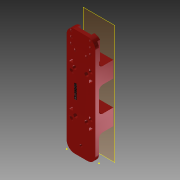
# Autodesk Inventor part: 150mm Link_V2 PART A
Saved by Autodesk Inventor 2015 (Build 190159000, 159)
## iProperties
Created: 2016-11-30
Part Number: 150mm Link_V2 PART A
Material: Generic
Document SubType Name: Modeling
Designer: Rudge-Top
Density: 1 g/cm^3
Appearance: Orange-Red
Author: Rudge-Top
Autodesk Inventor part; units mm, degrees
ref_plane "YZ Plane" through (0, 0, 0) normal (1, 0, 0) x (0, 1, 0)
ref_plane "XZ Plane" through (0, 0, 0) normal (0, 1, 0) x (-1, 0, 0)
ref_plane "XY Plane" through (0, 0, 0) normal (0, 0, 1) x (1, 0, 0)
sketch "Sketch1" plane through (0, 0, 0) normal (1, 0, 0) x (0, 1, 0)
  line L0 (120, 0) -> (150, 0)
  line L1 (150, 0) -> (150, -40)
  line L2 (150, -40) -> (120, -40)
  line L3 (150, 5) -> (0, 5)
  line L4 (0, -45) -> (150, -45)
  line L5 (150, 0) -> (150, 5)
  line L6 (150, -40) -> (150, -45)
  line L7 (0, -40) -> (0, -45)
  line L8 (0, 0) -> (0, 5)
  line L9 (115, -5) -> (115, -35)
  arc A0 (120, 0) -> (115, -5) centre (120, -5) ccw
  arc A1 (115, -35) -> (120, -40) centre (120, -35) ccw
  line L10 (87.5, 0) -> (62.5, 0)
  line L11 (57.5, -5) -> (57.5, -35)
  line L12 (62.5, -40) -> (87.5, -40)
  line L13 (92.5, -35) -> (92.5, -5)
  arc A2 (87.5, -40) -> (92.5, -35) centre (87.5, -35) ccw
  arc A3 (57.5, -35) -> (62.5, -40) centre (62.5, -35) ccw
  arc A4 (62.5, 0) -> (57.5, -5) centre (62.5, -5) ccw
  arc A5 (92.5, -5) -> (87.5, 0) centre (87.5, -5) ccw
  line L14 (0, 0) -> (30, 0)
  line L15 (35, -5) -> (35, -35)
  line L16 (30, -40) -> (0, -40)
  arc A6 (35, -5) -> (30, 0) centre (30, -5) ccw
  arc A7 (30, -40) -> (35, -35) centre (30, -35) ccw
  point P0 (57.5, -40)
  point P1 (92.5, -40)
  point P2 (35, 0)
  dimension "d1" = 150
  dimension "d2" = 40
  dimension "d3" = 90
  dimension "d4" = 5
  dimension "d5" = 35
  dimension "d6" = 5
  dimension "d7" = 35
  dimension "d8" = 5
  dimension "d9" = 22.5
  dimension "d10" = 5
  dimension "d11" = 35
  dimension "d12" = 5
  constraints: 34 end point, 16 point on circle, 16 tangent, 9 point on line, 8 centre point, 8 perpendicular, 5 equal radius, 3 horizontal, 2 parallel
  measures "d1" distance of L8.start L0.end
  measures "d2" distance of L0.end L1.end
  measures "d3" angle of L0 L1
  measures "d4" distance between parallel lines of L0 L3
  measures "d5" distance between parallel lines of L1 L9
  measures "d6" radius of A0
  measures "d7" distance of point (92.5, -40) point (57.5, -40)
  measures "d8" distance between parallel lines of L3 L10
  measures "d9" distance between parallel lines of L13 L9
  measures "d10" radius of A2
  measures "d11" distance of L8.start point (35, 0)
  measures "d12" radius of A6
extrude "Extrusion1" add sketch "Sketch1" along normal blind 40 contours A0 L9 A1 L2 L6 L4 L7 L16 A7 L15 A6 L14 L8 L3 L5 L0
sketch "Sketch2" plane through (40, 0, 0) normal (1, 0, 0) x (0, 0, -1)
  arc A0 (35, 57.5) -> (40, 62.5) centre (35, 62.5) ccw projected
  line L0 (35, 57.5) -> (5, 57.5) projected
  arc A1 (0, 62.5) -> (5, 57.5) centre (5, 62.5) ccw projected
  line L1 (0, 62.5) -> (0, 87.5) projected
  arc A2 (5, 92.5) -> (0, 87.5) centre (5, 87.5) ccw projected
  line L2 (5, 92.5) -> (35, 92.5) projected
  arc A3 (40, 87.5) -> (35, 92.5) centre (35, 87.5) ccw projected
  line L3 (40, 87.5) -> (40, 62.5) projected
  line L4 (0, 0) -> (0, 30) projected
  arc A4 (5, 35) -> (0, 30) centre (5, 30) ccw projected
  line L5 (5, 35) -> (35, 35) projected
  arc A5 (40, 30) -> (35, 35) centre (35, 30) ccw projected
  line L6 (40, 30) -> (40, 0) projected
  line L7 (40, 0) -> (45, 0) projected
  line L8 (45, 0) -> (45, 150) projected
  line L9 (45, 150) -> (40, 150) projected
  line L10 (40, 150) -> (40, 120) projected
  arc A6 (35, 115) -> (40, 120) centre (35, 120) ccw projected
  line L11 (35, 115) -> (5, 115) projected
  arc A7 (0, 120) -> (5, 115) centre (5, 120) ccw projected
  line L12 (0, 120) -> (0, 150) projected
  line L13 (0, 150) -> (-5, 150) projected
  line L14 (-5, 150) -> (-5, 0) projected
  line L15 (-5, 0) -> (0, 0) projected
  circle A8 centre (35, 45.25) radius 2.5
  circle A9 centre (25, 45.25) radius 2.5
  circle A10 centre (15, 45.25) radius 2.5
  circle A11 centre (5, 45.25) radius 2.5
  circle A12 centre (35, 104.75) radius 2.5
  circle A13 centre (25, 104.75) radius 2.5
  circle A14 centre (15, 104.75) radius 2.5
  circle A15 centre (5, 104.75) radius 2.5
  dimension "d15" = 5
  dimension "d16" = 5
  dimension "d17" = 5
  dimension "d18" = 5
  dimension "d19" = 10
  dimension "d20" = 20
  dimension "d21" = 30
  dimension "d22" = 40
  dimension "d23" = 5
  dimension "d24" = 5
  dimension "d25" = 5
  dimension "d26" = 5
  dimension "d27" = 12.25
  dimension "d28" = 12.25
  dimension "d29" = 12.25
  dimension "d30" = 12.25
  dimension "d31" = 12.25
  dimension "d32" = 12.25
  dimension "d33" = 12.25
  dimension "d34" = 12.25
  constraints: 8 centre point
  measures "d15" diameter of A8
  measures "d16" diameter of A9
  measures "d17" diameter of A10
  measures "d18" diameter of A11
  measures "d19" distance from line of L14 A11.centre
  measures "d20" distance from line of A10.centre L14
  measures "d21" distance from line of A9.centre L14
  measures "d22" distance from line of A8.centre L14
  measures "d23" diameter of A12
  measures "d24" diameter of A13
  measures "d25" diameter of A14
  measures "d26" diameter of A15
  measures "d27" distance from line of A12.centre L2
  measures "d28" distance from line of L2 A13.centre
  measures "d29" distance from line of L2 A14.centre
  measures "d30" distance from line of L2 A15.centre
  measures "d31" distance from line of A8.centre L0
  measures "d32" distance from line of A9.centre L0
  measures "d33" distance from line of A10.centre L0
  measures "d34" distance from line of A11.centre L0
fillet "Fillet1" radius 11 8 edges at (40, 0, 2.5) (0, 0, 2.5) (40, 0, -42.5) (0, 0, -42.5) (40, 150, 2.5) (40, 150, -42.5) (0, 150, -42.5) (0, 150, 2.5)
sketch "Sketch3" plane through (0, 11, -45) normal (0, 0, -1) x (-1, 0, 0)
  line L0 (0, 51.5) -> (-40, 51.5) projected
  arc A0 (0, 128) -> (-11, 139) centre (-11, 128) ccw projected
  line L1 (-11, 139) -> (-29, 139) projected
  arc A1 (-29, 139) -> (-40, 128) centre (-29, 128) ccw projected
  line L2 (-40, 0) -> (-40, 128) projected
  arc A2 (-40, 0) -> (-29, -11) centre (-29, 0) ccw projected
  line L3 (-11, -11) -> (-29, -11) projected
  arc A3 (-11, -11) -> (0, 0) centre (-11, 0) ccw projected
  line L4 (0, 0) -> (0, 128) projected
  line L5 (-40, 51.5) -> (-40, 46.5) projected
  line L6 (-40, 46.5) -> (-40, 51.5) projected
  line L7 (-40, 51.5) -> (-40, 76.5) projected
  line L8 (-40, 76.5) -> (-40, 81.5) projected
  line L9 (-40, 81.5) -> (-40, 76.5) projected
  line L10 (-40, 76.5) -> (-40, 51.5) projected
  line L11 (-40, 128) -> (-40, 109) projected
  line L12 (-40, 109) -> (-40, 104) projected
  line L13 (-40, 104) -> (-40, 109) projected
  line L14 (-40, 109) -> (-40, 128) projected
  line L15 (-40, 128) -> (-40, 0) projected
  line L16 (-40, 0) -> (-40, 19) projected
  line L17 (-40, 19) -> (-40, 24) projected
  line L18 (-40, 24) -> (-40, 19) projected
  line L19 (-40, 19) -> (-40, 0) projected
  line L20 (-40, 0) -> (-40, 128) projected
  line L21 (-9, 26.5) -> (-31, 26.5)
  line L22 (-36, 31.5) -> (-36, 39)
  line L23 (-31, 44) -> (-9, 44)
  line L24 (-4, 39) -> (-4, 31.5)
  arc A4 (-36, 31.5) -> (-31, 26.5) centre (-31, 31.5) ccw
  arc A5 (-31, 44) -> (-36, 39) centre (-31, 39) ccw
  arc A6 (-4, 39) -> (-9, 44) centre (-9, 39) ccw
  arc A7 (-9, 26.5) -> (-4, 31.5) centre (-9, 31.5) ccw
  line L25 (-9, 84) -> (-31, 84)
  line L26 (-36, 89) -> (-36, 96.5)
  line L27 (-31, 101.5) -> (-9, 101.5)
  line L28 (-4, 96.5) -> (-4, 89)
  arc A8 (-36, 89) -> (-31, 84) centre (-31, 89) ccw
  arc A9 (-31, 101.5) -> (-36, 96.5) centre (-31, 96.5) ccw
  arc A10 (-4, 96.5) -> (-9, 101.5) centre (-9, 96.5) ccw
  arc A11 (-9, 84) -> (-4, 89) centre (-9, 89) ccw
  circle A12 centre (-27.6928, 35.25) radius 1.5
  circle A13 centre (-12.3072, 35.25) radius 1.5
  circle A14 centre (-27.6928, 92.75) radius 1.5
  circle A15 centre (-11, 92.75) radius 1.5
  line L29 (-36, 39) -> (-33, 39)
  line L30 (-31, 41) -> (-31, 44)
  line L31 (-33, 31.5) -> (-36, 31.5)
  line L32 (-31, 29.5) -> (-31, 26.5)
  arc A16 (-31, 29.5) -> (-33, 31.5) centre (-33, 29.5) ccw
  arc A17 (-33, 39) -> (-31, 41) centre (-33, 41) ccw
  line L33 (-7, 31.5) -> (-4, 31.5)
  line L34 (-9, 29.5) -> (-9, 26.5)
  line L35 (0, 128) -> (0, 0) projected
  line L36 (-7, 39) -> (-4, 39)
  line L37 (-9, 41) -> (-9, 44)
  arc A18 (-7, 31.5) -> (-9, 29.5) centre (-7, 29.5) ccw
  arc A19 (-9, 41) -> (-7, 39) centre (-7, 41) ccw
  line L38 (-36, 89) -> (-33, 89)
  line L39 (-31, 87) -> (-31, 84)
  line L40 (-7.5, 89) -> (-4, 89)
  line L41 (-9.5, 87) -> (-9.5, 84)
  line L42 (-4, 96.5) -> (-7, 96.5)
  line L43 (-9, 98.5) -> (-9, 101.5)
  line L44 (-31, 101.5) -> (-31, 98.5)
  line L45 (-33, 96.5) -> (-36, 96.5)
  arc A20 (-31, 87) -> (-33, 89) centre (-33, 87) ccw
  arc A21 (-33, 96.5) -> (-31, 98.5) centre (-33, 98.5) ccw
  arc A22 (-9, 98.5) -> (-7, 96.5) centre (-7, 98.5) ccw
  arc A23 (-7.5, 89) -> (-9.5, 87) centre (-7.5, 87) ccw
  point P0 (0, -11)
  point P1 (-40, 91.25)
  point P2 (-40, 96.25)
  point P3 (-40, 91.25)
  point P4 (-40, 96.25)
  point P5 (-40, 31.75)
  point P6 (-40, 36.75)
  point P7 (-40, 31.75)
  point P8 (-40, 36.75)
  point P9 (-40, 31.75)
  point P10 (-40, 36.75)
  point P11 (-40, 31.75)
  point P12 (-40, 36.75)
  point P13 (-40, 91.25)
  point P14 (-40, 96.25)
  point P15 (-40, 91.25)
  point P16 (-40, 96.25)
  point P17 (-36, 44)
  point P18 (-36, 26.5)
  point P19 (-4, 44)
  dimension "d38" = 32
  dimension "d39" = 17.5
  dimension "d40" = 55
  dimension "d41" = 5
  dimension "d42" = 5
  dimension "d43" = 55
  dimension "d73" = 4
  dimension "d74" = 4
  dimension "d75" = 32
  dimension "d120" = 3
  dimension "d121" = 3
  dimension "d122" = 3
  dimension "d123" = 3
  dimension "d124" = 2
  dimension "d125" = 2
  dimension "d126" = 2
  constraints: 48 end point, 32 point on circle, 32 tangent, 22 point on line, 20 centre point, 11 equal radius, 11 perpendicular, 6 horizontal, 5 parallel, 2 vertical
  measures "d38" distance of point (-36, 44) point (-4, 44)
  measures "d39" distance of point (-36, 26.5) point (-36, 44)
  measures "d40" distance between parallel lines of L3 L23
  measures "d41" radius of A4
  measures "d42" radius of A8
  measures "d43" distance between parallel lines of L1 L25
  measures "d73" distance between parallel lines of L4 L24
  measures "d74" distance between parallel lines of L4 L28
  measures "d75" distance between parallel lines of L28 L26
  measures "d120" diameter of A12
  measures "d121" diameter of A13
  measures "d122" diameter of A14
  measures "d123" diameter of A15
  measures "d124" radius of A16
  measures "d125" radius of A18
  measures "d126" radius of A20
sketch "Sketch4" plane through (0, 11, 5) normal (0, 0, 1) x (1, 0, 0)
  line L0 (13.7515, 74.4502) -> (13.7515, 54.5408) construction
  line L1 (13.7515, 54.5408) -> (10.1902, 54.5408) construction
  line L2 (10.1902, 54.5408) -> (10.1902, 74.4502) construction
  line L3 (10.1902, 74.4502) -> (13.7515, 74.4502) construction
  point P0 (0, -11)
  constraints: 2 other
sketch "Sketch5" plane through (40, 0, 0) normal (1, 0, 0) x (0, 0, -1)
  point P0 (0, 0)
sketch "Sketch6" plane through (0, 30, -40) normal (0, 0, 1) x (1, 0, 0)
  arc A0 (0, -19) -> (11, -30) centre (11, -19) ccw projected
  line L0 (11, -30) -> (29, -30) projected
  arc A1 (29, -30) -> (40, -19) centre (29, -19) ccw projected
  line L1 (40, 0) -> (40, -19) projected
  line L2 (0, 0) -> (40, 0) projected
  line L3 (0, 0) -> (0, -19) projected
  arc A2 (12, -23.5498) -> (12, -8.4502) centre (20, -16) ccw
  line L4 (12, -34.5405) -> (12, 2.5405)
  arc A3 (12, -26.247) -> (12, -5.753) centre (20, -16) ccw
  point P0 (0, -30)
  point P1 (12, -16.0119)
  point P2 (20.0119, -24)
  point P3 (28, -15.9881)
  point P4 (19.9881, -8)
  dimension "d46" = 22
  dimension "d47" = 14
  dimension "d48" = 8
  dimension "d51" = 360
  dimension "d71" = 20
  dimension "d115" = 13
  constraints: 5 point on line, 4 point on circle, 2 centre point, 2 end point, 1 coincident, 1 vertical, 5 other
  measures "d46" diameter of A2
  measures "d47" distance from line of L0 A2.centre
  measures "d48" distance of A2.centre point (12, -16.012)
  measures "d71" distance from line of L3 A2.centre
  measures "d115" radius of A3
hole "Hole1" at (20.0119, 6, -40) at (12, 13.9881, -40) at (28, 14.0119, -40) at (19.9881, 22, -40) direction (0, 0, -1) diameter 2 end through all
extrude "Extrusion4" add sketch "Sketch6" along normal blind 4 contours L4 A2 A3
sketch "Sketch7" plane through (0, 11, 5) normal (0, 0, 1) x (1, 0, 0)
  arc A0 (11, 139) -> (0, 128) centre (11, 128) ccw projected
  line L0 (0, 128) -> (0, 0) projected
  arc A1 (0, 0) -> (11, -11) centre (11, 0) ccw projected
  line L1 (11, -11) -> (29, -11) projected
  arc A2 (29, -11) -> (40, 0) centre (29, 0) ccw projected
  line L2 (40, 128) -> (40, 0) projected
  arc A3 (40, 128) -> (29, 139) centre (29, 128) ccw projected
  line L3 (11, 139) -> (29, 139) projected
  circle A4 centre (28, 3.0119) radius 1 projected
  circle A5 centre (19.9881, 11) radius 1 projected
  circle A6 centre (12, 2.9881) radius 1 projected
  circle A7 centre (20.0119, -5) radius 1 projected
  point P0 (0, -11)
  point P1 (20, 3)
  dimension "d63" = 8
  dimension "d72" = 8
  measures "d63" distance of point (20, 3) A4.centre
  measures "d72" distance of A5.centre point (20, 3)
hole "Hole2" at (20, 14, 5) direction (0, 0, -1) diameter 4 end through all
sketch "Sketch8" plane through (0, 120, -40) normal (0, 0, 1) x (1, 0, 0)
  arc A0 (11, 30) -> (0, 19) centre (11, 19) ccw projected
  line L0 (0, 19) -> (0, 0) projected
  line L1 (0, 0) -> (40, 0) projected
  line L2 (40, 19) -> (40, 0) projected
  arc A1 (40, 19) -> (29, 30) centre (29, 19) ccw projected
  line L3 (11, 30) -> (29, 30) projected
  line L4 (11, 30) -> (29, 30) projected
  line L5 (20, 10) -> (20, 0)
  line L6 (29, 30) -> (29.5, 30)
  arc A2 (40, 19) -> (29, 30) centre (29, 19) ccw projected
  line L7 (29.5, 30) -> (29.5, 10)
  line L8 (29.5, 10) -> (24, 10)
  line L9 (0, 0) -> (40, 0) projected
  line L10 (37.5, 0) -> (37.5, 25.9821)
  arc A3 (37.5, 25.9821) -> (29.5, 30) centre (28.9549, 18.9413) ccw
  line L11 (24, 10) -> (24, 0)
  arc A4 (11, 30) -> (0, 19) centre (11, 19) ccw
  line L12 (10.5, 30) -> (10.5, 10)
  line L13 (10.5, 10) -> (16, 10)
  line L14 (2.5, 0) -> (2.5, 25.9821)
  arc A5 (10.5, 30) -> (2.5, 25.9821) centre (11.0451, 18.9413) ccw
  line L15 (16, 10) -> (16, 0)
  line L16 (37.5, 0) -> (24, 0)
  line L17 (31, -7.5) -> (9, -7.5) projected
  line L18 (16, 0) -> (2.5, 0)
  arc A6 (10.5, 30) -> (2.5, 25.9821) centre (11.0451, 18.9413) ccw
  point P0 (0, -120)
  dimension "d77" = 10
  dimension "d78" = 9.5
  dimension "d80" = 17.5
  dimension "d81" = 4
  constraints: 24 end point, 9 point on circle, 8 symmetric about line, 4 centre point, 3 point on line, 3 vertical, 2 tangent, 1 collinear, 1 midpoint, 1 parallel, 1 perpendicular, 2 other
  measures "d77" distance between parallel lines of L8 L1
  measures "d78" distance between parallel lines of L5 L7
  measures "d80" distance between parallel lines of L10 L5
  measures "d81" distance between parallel lines of L5 L11
extrude "Extrusion5" add sketch "Sketch8" along normal blind 4 contours A5 L12 A0 | A0 L12 L13 L15 L1 L14 | L10 L1 L11 L8 L7 A1 | L7 A3 A1
ref_plane "Work Plane1" through (0, 11, -20) normal (0, 0, 1) x (1, 0, 0)
mirror "Mirror1" about plane through (0, 11, -20) normal (0, 0, 1) of "Extrusion5"
sketch "Sketch9" plane through (0, 11, -45) normal (0, 0, -1) x (-1, 0, 0)
  circle A0 centre (-20, 3) radius 2 projected
  circle A1 centre (-28, 3.0119) radius 1 projected
  circle A2 centre (-20.0119, -5) radius 1 projected
  circle A3 centre (-12, 2.9881) radius 1 projected
  circle A4 centre (-19.9881, 11) radius 1 projected
  arc A5 (0, 128) -> (-11, 139) centre (-11, 128) ccw projected
  line L0 (-11, 139) -> (-29, 139) projected
  arc A6 (-29, 139) -> (-40, 128) centre (-29, 128) ccw projected
  line L1 (-40, 0) -> (-40, 128) projected
  arc A7 (-40, 0) -> (-29, -11) centre (-29, 0) ccw projected
  line L2 (-11, -11) -> (-29, -11) projected
  arc A8 (-11, -11) -> (0, 0) centre (-11, 0) ccw projected
  line L3 (0, 0) -> (0, 128) projected
  arc A9 (-29.5, 139) -> (-37.5, 134.9821) centre (-28.9549, 127.9413) ccw projected
  line L4 (-37.5, 109) -> (-37.5, 134.9821) projected
  line L5 (-24, 109) -> (-37.5, 109) projected
  line L6 (-24, 119) -> (-24, 109) projected
  line L7 (-29.5, 119) -> (-24, 119) projected
  line L8 (-29.5, 139) -> (-29.5, 119) projected
  line L9 (-2.5, 109) -> (-16, 109) projected
  line L10 (-2.5, 134.9821) -> (-2.5, 109) projected
  arc A10 (-2.5, 134.9821) -> (-10.5, 139) centre (-11.0451, 127.9413) ccw projected
  line L11 (-10.5, 119) -> (-10.5, 139) projected
  line L12 (-16, 119) -> (-10.5, 119) projected
  line L13 (-16, 109) -> (-16, 119) projected
  line L14 (-16, 109) -> (-24, 109)
  line L15 (-20, 109) -> (-20, 113.033)
  point P0 (0, -11)
  point P1 (-28, 114)
  point P2 (-12, 114)
  point P3 (-6.5, 119.25)
  point P4 (-6.5, 127.25)
  point P5 (-6.5, 135.25)
  point P6 (-33.5, 119.25)
  point P7 (-33.5, 127.25)
  point P8 (-33.5, 135.25)
  dimension "d84" = 4
  dimension "d85" = 16
  dimension "d86" = 5
  dimension "d87" = 5.25
  dimension "d88" = 8
  dimension "d89" = 8
  dimension "d90" = 4
  dimension "d91" = 4
  dimension "d92" = 4
  constraints: 4 end point, 3 symmetric about line, 1 horizontal, 1 midpoint, 1 vertical
  measures "d84" distance from line of L6 point (-28, 114)
  measures "d85" distance of point (-12, 114) point (-28, 114)
  measures "d86" distance from line of point (-28, 114) L5
  measures "d87" vertical distance of point (-12, 114) point (-6.5, 119.25)
  measures "d88" distance of point (-6.5, 127.25) point (-6.5, 119.25)
  measures "d89" distance of point (-6.5, 127.25) point (-6.5, 135.25)
  measures "d90" distance from line of L10 point (-6.5, 119.25)
  measures "d91" distance from line of L10 point (-6.5, 127.25)
  measures "d92" distance from line of L10 point (-6.5, 135.25)
hole "Hole3" at (33.5, 146.25, -45) at (33.5, 138.25, -45) at (33.5, 130.25, -45) at (28, 125, -45) at (12, 125, -45) at (6.5, 130.25, -45) at (6.5, 138.25, -45) at (6.5, 146.25, -45) direction (0, 0, 1) diameter 2 end through all
sketch "Sketch10" plane through (0, 11, 5) normal (0, 0, 1) x (1, 0, 0)
  circle A0 centre (6.5, 127.25) radius 1 projected
  circle A1 centre (12, 114) radius 1 projected
  circle A2 centre (33.5, 119.25) radius 1 projected
  circle A3 centre (33.5, 135.25) radius 1 projected
  circle A4 centre (33.5, 127.25) radius 1 projected
  circle A5 centre (28, 114) radius 1 projected
  circle A6 centre (6.5, 119.25) radius 1 projected
  circle A7 centre (6.5, 135.25) radius 1 projected
  circle A8 centre (20, 3) radius 2 projected
  arc A9 (11, 139) -> (0, 128) centre (11, 128) ccw projected
  line L0 (0, 128) -> (0, 0) projected
  arc A10 (0, 0) -> (11, -11) centre (11, 0) ccw projected
  line L1 (11, -11) -> (29, -11) projected
  arc A11 (29, -11) -> (40, 0) centre (29, 0) ccw projected
  line L2 (40, 128) -> (40, 0) projected
  arc A12 (40, 128) -> (29, 139) centre (29, 128) ccw projected
  line L3 (11, 139) -> (29, 139) projected
  line L4 (28, 111.6906) -> (26, 112.8453)
  line L5 (26, 112.8453) -> (26, 115.1547)
  line L6 (26, 115.1547) -> (28, 116.3094)
  line L7 (28, 116.3094) -> (30, 115.1547)
  line L8 (30, 115.1547) -> (30, 112.8453)
  line L9 (30, 112.8453) -> (28, 111.6906)
  line L10 (12, 111.6906) -> (10, 112.8453)
  line L11 (10, 112.8453) -> (10, 115.1547)
  line L12 (10, 115.1547) -> (12, 116.3094)
  line L13 (12, 116.3094) -> (14, 115.1547)
  line L14 (14, 115.1547) -> (14, 112.8453)
  line L15 (14, 112.8453) -> (12, 111.6906)
  line L16 (6.5, 116.9406) -> (4.5, 118.0953)
  line L17 (4.5, 118.0953) -> (4.5, 120.4047)
  line L18 (4.5, 120.4047) -> (6.5, 121.5594)
  line L19 (6.5, 121.5594) -> (8.5, 120.4047)
  line L20 (8.5, 120.4047) -> (8.5, 118.0953)
  line L21 (8.5, 118.0953) -> (6.5, 116.9406)
  line L22 (6.5, 124.9406) -> (4.5, 126.0953)
  line L23 (4.5, 126.0953) -> (4.5, 128.4047)
  line L24 (4.5, 128.4047) -> (6.5, 129.5594)
  line L25 (6.5, 129.5594) -> (8.5, 128.4047)
  line L26 (8.5, 128.4047) -> (8.5, 126.0953)
  line L27 (8.5, 126.0953) -> (6.5, 124.9406)
  circle A13 centre (6.5, 127.25) radius 1
  circle A14 centre (6.5, 119.25) radius 1
  circle A15 centre (12, 114) radius 1
  circle A16 centre (28, 114) radius 1
  line L28 (33.5, 132.9406) -> (31.5, 134.0953)
  line L29 (31.5, 134.0953) -> (31.5, 136.4047)
  line L30 (31.5, 136.4047) -> (33.5, 137.5594)
  line L31 (33.5, 137.5594) -> (35.5, 136.4047)
  line L32 (35.5, 136.4047) -> (35.5, 134.0953)
  line L33 (35.5, 134.0953) -> (33.5, 132.9406)
  line L34 (6.5, 137.5594) -> (8.5, 136.4047)
  line L35 (8.5, 136.4047) -> (8.5, 134.0953)
  line L36 (8.5, 134.0953) -> (6.5, 132.9406)
  line L37 (6.5, 132.9406) -> (4.5, 134.0953)
  line L38 (4.5, 134.0953) -> (4.5, 136.4047)
  line L39 (4.5, 136.4047) -> (6.5, 137.5594)
  circle A17 centre (6.5, 135.25) radius 1
  circle A18 centre (33.5, 135.25) radius 1
  line L40 (33.5, 129.5594) -> (35.5, 128.4047)
  line L41 (35.5, 128.4047) -> (35.5, 126.0953)
  line L42 (35.5, 126.0953) -> (33.5, 124.9406)
  line L43 (33.5, 124.9406) -> (31.5, 126.0953)
  line L44 (31.5, 126.0953) -> (31.5, 128.4047)
  line L45 (31.5, 128.4047) -> (33.5, 129.5594)
  line L46 (33.5, 121.5594) -> (35.5, 120.4047)
  line L47 (35.5, 120.4047) -> (35.5, 118.0953)
  line L48 (35.5, 118.0953) -> (33.5, 116.9406)
  line L49 (33.5, 116.9406) -> (31.5, 118.0953)
  line L50 (31.5, 118.0953) -> (31.5, 120.4047)
  line L51 (31.5, 120.4047) -> (33.5, 121.5594)
  circle A19 centre (33.5, 127.25) radius 1
  circle A20 centre (33.5, 119.25) radius 1
  point P0 (0, -11)
  dimension "d102" = 4
  dimension "d103" = 4
  dimension "d104" = 4
  dimension "d105" = 4
  dimension "d111" = 4
  dimension "d112" = 4
  dimension "d113" = 4
  dimension "d114" = 4
  constraints: 96 end point, 8 centre point, 7 coincident, 3 concentric, 52 other
  measures "d102" distance between parallel lines of L8 L5
  measures "d103" distance between parallel lines of L14 L11
  measures "d104" distance between parallel lines of L20 L17
  measures "d105" distance between parallel lines of L26 L23
  measures "d111" distance between parallel lines of L29 L32
  measures "d112" distance between parallel lines of L35 L38
  measures "d113" distance between parallel lines of L47 L50
  measures "d114" distance between parallel lines of L41 L44
extrude "Extrusion6" cut sketch "Sketch10" against normal blind 1.6 contours L4 L5 L6 L7 L8 L9 | L10 L11 L12 L13 L14 L15 | L16 L17 L18 L19 L20 L21 | L22 L23 L24 L25 L26 L27 | L28 L29 L30 L31 L32 L33 | L34 L35 L36 L37 L38 L39 | L40 L41 L42 L43 L44 L45 | L46 L47 L48 L49 L50 L51
mirror "Mirror2" about plane through (0, 11, -20) normal (0, 0, 1) of "Extrusion6"
sketch "Sketch11" plane through (40, 0, 0) normal (1, 0, 0) x (0, 0, -1)
  point P0 (0, 0)
sketch "Sketch12" plane through (0, 11, -20) normal (0, 0, 1) x (1, 0, 0)
  line L0 (42.278, 147.4022) -> (0, 147.4022)
  line L1 (0, 147.4022) -> (0, -18.4991)
  line L2 (0, -18.4991) -> (42.278, -18.4991)
  line L3 (42.278, -18.4991) -> (42.278, 147.4022)
  point P0 (0, -11)
  constraints: 8 end point, 2 parallel, 1 horizontal, 1 perpendicular
extrude "Extrusion7" cut sketch "Sketch12" against normal blind 83.025
extrude "Extrusion9" cut sketch "Sketch3" against normal blind 70 contours L34 A18 L33 A7 | A4 L31 A16 L32 | L36 A19 L37 A6 | A5 L30 A17 L29 | L25 L41 A23 L40 A11 | A8 L38 A20 L39 | L42 A22 L43 A10 | A9 L44 A21 L45 | A12 | A13 | A14 | A15
sketch "Sketch14" plane through (0, 11, 5) normal (0, 0, 1) x (1, 0, 0)
  line L0 (0, 19) -> (40, 19) projected
  circle A0 centre (27.6928, 35.25) radius 1.5 projected
  circle A1 centre (27.6928, 92.75) radius 1.5 projected
  line L1 (9, 101.5) -> (9, 98.5) projected
  arc A2 (7, 96.5) -> (9, 98.5) centre (7, 98.5) ccw projected
  line L2 (7, 96.5) -> (4, 96.5) projected
  arc A3 (9, 101.5) -> (4, 96.5) centre (9, 96.5) ccw projected
  line L3 (31, 84) -> (31, 87) projected
  arc A4 (33, 89) -> (31, 87) centre (33, 87) ccw projected
  line L4 (33, 89) -> (36, 89) projected
  arc A5 (31, 84) -> (36, 89) centre (31, 89) ccw projected
  arc A6 (7, 39) -> (9, 41) centre (7, 41) ccw projected
  line L5 (7, 39) -> (4, 39) projected
  arc A7 (9, 44) -> (4, 39) centre (9, 39) ccw projected
  line L6 (9, 44) -> (9, 41) projected
  arc A8 (33, 31.5) -> (31, 29.5) centre (33, 29.5) ccw projected
  line L7 (33, 31.5) -> (36, 31.5) projected
  arc A9 (31, 26.5) -> (36, 31.5) centre (31, 31.5) ccw projected
  line L8 (31, 26.5) -> (31, 29.5) projected
  line L9 (36, 39) -> (33, 39) projected
  arc A10 (31, 41) -> (33, 39) centre (33, 41) ccw projected
  line L10 (31, 41) -> (31, 44) projected
  arc A11 (36, 39) -> (31, 44) centre (31, 39) ccw projected
  arc A12 (9, 29.5) -> (7, 31.5) centre (7, 29.5) ccw projected
  line L11 (9, 29.5) -> (9, 26.5) projected
  arc A13 (4, 31.5) -> (9, 26.5) centre (9, 31.5) ccw projected
  line L12 (4, 31.5) -> (7, 31.5) projected
  arc A14 (31, 98.5) -> (33, 96.5) centre (33, 98.5) ccw projected
  line L13 (31, 98.5) -> (31, 101.5) projected
  arc A15 (36, 96.5) -> (31, 101.5) centre (31, 96.5) ccw projected
  line L14 (36, 96.5) -> (33, 96.5) projected
  line L15 (4, 89) -> (7.5, 89) projected
  arc A16 (9.5, 87) -> (7.5, 89) centre (7.5, 87) ccw projected
  line L16 (9.5, 87) -> (9.5, 84) projected
  line L17 (9.5, 84) -> (9, 84) projected
  arc A17 (4, 89) -> (9, 84) centre (9, 89) ccw projected
  circle A18 centre (11, 92.75) radius 1.5 projected
  circle A19 centre (12.3072, 35.25) radius 1.5 projected
  line L18 (31.5, 128.4047) -> (33.5, 129.5594) projected
  line L19 (33.5, 129.5594) -> (35.5, 128.4047) projected
  line L20 (35.5, 128.4047) -> (35.5, 126.0953) projected
  line L21 (35.5, 126.0953) -> (33.5, 124.9406) projected
  line L22 (33.5, 124.9406) -> (31.5, 126.0953) projected
  line L23 (31.5, 126.0953) -> (31.5, 128.4047) projected
  line L24 (35.5, 134.0953) -> (33.5, 132.9406) projected
  line L25 (33.5, 132.9406) -> (31.5, 134.0953) projected
  line L26 (31.5, 134.0953) -> (31.5, 136.4047) projected
  line L27 (31.5, 136.4047) -> (33.5, 137.5594) projected
  line L28 (33.5, 137.5594) -> (35.5, 136.4047) projected
  line L29 (35.5, 136.4047) -> (35.5, 134.0953) projected
  line L30 (4.5, 120.4047) -> (6.5, 121.5594) projected
  line L31 (6.5, 121.5594) -> (8.5, 120.4047) projected
  line L32 (8.5, 120.4047) -> (8.5, 118.0953) projected
  line L33 (8.5, 118.0953) -> (6.5, 116.9406) projected
  line L34 (6.5, 116.9406) -> (4.5, 118.0953) projected
  line L35 (4.5, 118.0953) -> (4.5, 120.4047) projected
  line L36 (26, 115.1547) -> (28, 116.3094) projected
  line L37 (28, 116.3094) -> (30, 115.1547) projected
  line L38 (30, 115.1547) -> (30, 112.8453) projected
  line L39 (30, 112.8453) -> (28, 111.6906) projected
  line L40 (28, 111.6906) -> (26, 112.8453) projected
  line L41 (26, 112.8453) -> (26, 115.1547) projected
  line L42 (10, 115.1547) -> (12, 116.3094) projected
  line L43 (12, 116.3094) -> (14, 115.1547) projected
  line L44 (14, 115.1547) -> (14, 112.8453) projected
  line L45 (14, 112.8453) -> (12, 111.6906) projected
  line L46 (12, 111.6906) -> (10, 112.8453) projected
  line L47 (10, 112.8453) -> (10, 115.1547) projected
  line L48 (4.5, 128.4047) -> (6.5, 129.5594) projected
  line L49 (6.5, 129.5594) -> (8.5, 128.4047) projected
  line L50 (8.5, 128.4047) -> (8.5, 126.0953) projected
  line L51 (8.5, 126.0953) -> (6.5, 124.9406) projected
  line L52 (6.5, 124.9406) -> (4.5, 126.0953) projected
  line L53 (4.5, 126.0953) -> (4.5, 128.4047) projected
  line L54 (4.5, 136.4047) -> (6.5, 137.5594) projected
  line L55 (6.5, 137.5594) -> (8.5, 136.4047) projected
  line L56 (8.5, 136.4047) -> (8.5, 134.0953) projected
  line L57 (8.5, 134.0953) -> (6.5, 132.9406) projected
  line L58 (6.5, 132.9406) -> (4.5, 134.0953) projected
  line L59 (4.5, 134.0953) -> (4.5, 136.4047) projected
  line L60 (31.5, 120.4047) -> (33.5, 121.5594) projected
  line L61 (33.5, 121.5594) -> (35.5, 120.4047) projected
  line L62 (35.5, 120.4047) -> (35.5, 118.0953) projected
  line L63 (35.5, 118.0953) -> (33.5, 116.9406) projected
  line L64 (33.5, 116.9406) -> (31.5, 118.0953) projected
  line L65 (31.5, 118.0953) -> (31.5, 120.4047) projected
  circle A20 centre (20, 3) radius 2 projected
  arc A21 (11, 139) -> (0, 128) centre (11, 128) ccw projected
  line L66 (0, 128) -> (0, 0) projected
  arc A22 (0, 0) -> (11, -11) centre (11, 0) ccw projected
  line L67 (11, -11) -> (29, -11) projected
  arc A23 (29, -11) -> (40, 0) centre (29, 0) ccw projected
  line L68 (40, 128) -> (40, 0) projected
  arc A24 (40, 128) -> (29, 139) centre (29, 128) ccw projected
  line L69 (11, 139) -> (29, 139) projected
  circle A25 centre (12.3072, 35.25) radius 1.5 projected
  line L70 (15.4826, 35.25) -> (13.8949, 32.5)
  line L71 (13.8949, 32.5) -> (10.7195, 32.5)
  line L72 (10.7195, 32.5) -> (9.1318, 35.25)
  line L73 (9.1318, 35.25) -> (10.7195, 38)
  line L74 (10.7195, 38) -> (13.8949, 38)
  line L75 (13.8949, 38) -> (15.4826, 35.25)
  line L76 (24.5174, 92.75) -> (26.1051, 95.5)
  line L77 (26.1051, 95.5) -> (29.2805, 95.5)
  line L78 (29.2805, 95.5) -> (30.8682, 92.75)
  line L79 (30.8682, 92.75) -> (29.2805, 90)
  line L80 (29.2805, 90) -> (26.1051, 90)
  line L81 (26.1051, 90) -> (24.5174, 92.75)
  circle A26 centre (27.6928, 35.25) radius 2.75
  circle A27 centre (11, 92.75) radius 2.75
  point P0 (0, -11)
  dimension "d129" = 5.5
  dimension "d130" = 5.5
  dimension "d131" = 5.5
  dimension "d132" = 5.5
  constraints: 24 end point, 4 coincident, 2 centre point, 26 other
  measures "d129" distance between parallel lines of L71 L74
  measures "d130" diameter of A26
  measures "d131" distance between parallel lines of L80 L77
  measures "d132" diameter of A27
extrude "Extrusion10" cut sketch "Sketch14" against normal blind 15 contours A1 | L70 L71 L72 L73 L74 L75 | L76 L77 L78 L79 L80 L81 | A26 | A27
body "Solid1"
